Autodesk Inventor part; units mm, degrees
(part 2 of 2)
sketch "Эскиз15" plane through (8.25, 13, 36.2214) normal (0, 0, 1) x (1, 0, 0)
  line L0 (0, 4.5) -> (0, 8)
  line L1 (0, 8) -> (-1, 8)
  line L2 (0, 0) -> (0, 4.5) projected
  line L3 (0, 4.5) -> (-3, 4.5)
  line L4 (-3.75, 4.5) -> (4.75, 4.5) projected
  line L5 (-1, 8) -> (-3, 4.5)
  line L6 (-3.75, 0) -> (-12.75, 0) construction
  line L7 (-8.25, 0) -> (-8.25, 4.5) construction
  line L8 (-12.75, 4.5) -> (-3.75, 4.5) construction
  line L9 (-16.5, 4.5) -> (-16.5, 8)
  line L10 (-16.5, 8) -> (-15.5, 8)
  line L11 (-16.5, 4.5) -> (-13.5, 4.5)
  line L12 (-15.5, 8) -> (-13.5, 4.5)
  point P0 (-8.25, -13)
  dimension "d200" = 3.5
  dimension "d201" = 1
  dimension "d202" = 3
  constraints: 18 end point, 4 symmetric about line, 2 midpoint, 1 perpendicular, 1 point on line, 1 vertical
  measures "d200" distance of L0.start L0.end
  measures "d201" distance of L0.end L1.end
  measures "d202" distance of L0.start L3.end
extrude "Выдавливание14" add sketch "Эскиз15" along normal blind 25.5
sketch "Эскиз16" plane through (0, 13, 0) normal (0, 1, 0) x (1, 0, 0)
  line L0 (14.893, -63.5381) -> (15, -63.3086) projected
  arc A0 (14.893, -63.5381) -> (13, -62.9053) centre (0, -104.941) ccw projected
  line L1 (13, -62.9053) -> (13, -48.5381) projected
  line L2 (15, -48.5381) -> (13, -48.5381) projected
  line L3 (15, -48.5381) -> (15, -63.3086) projected
  arc A1 (-13, -62.9053) -> (-14.893, -63.5381) centre (0, -104.941) ccw projected
  line L4 (-15, -63.3086) -> (-14.893, -63.5381) projected
  line L5 (-15, -63.3086) -> (-15, -48.5381) projected
  line L6 (-13, -48.5381) -> (-15, -48.5381) projected
  line L7 (-13, -48.5381) -> (-13, -62.9053) projected
  line L8 (8.25, -30.9214) -> (-8.25, -30.9214) projected
  point P0 (0, 0)
extrude "Выдавливание15" add sketch "Эскиз16" along normal blind 7
sketch "Эскиз17" plane through (0, 13, 0) normal (0, 1, 0) x (1, 0, 0)
  arc A0 (13, -62.9053) -> (8.25, -61.7214) centre (0, -104.941) ccw projected
  line L0 (11.5, -48.5381) -> (11.5, -66.0381) projected
  line L1 (8.25, -36.2214) -> (8.25, -61.7214) projected
  line L2 (11.5, -48.5381) -> (13, -48.5381) projected
  line L3 (11.5, -48.5381) -> (8.25, -48.5381)
  line L4 (0, -67.941) -> (0, -60.941) construction
  line L5 (-11.5, -48.5381) -> (-8.25, -48.5381)
  arc A1 (-8.25, -61.7214) -> (-13, -62.9053) centre (0, -104.941) ccw projected
  line L6 (-8.25, -36.2214) -> (-8.25, -61.7214) projected
  line L7 (-11.5, -48.5381) -> (-11.5, -66.0381) projected
  line L8 (13, -48.5381) -> (13, -62.9053) projected
  line L9 (15, -48.5381) -> (13, -48.5381) projected
  line L10 (15, -63.3086) -> (15, -48.5381) projected
  line L11 (14.893, -63.5381) -> (15, -63.3086) projected
  arc A2 (14.893, -63.5381) -> (13, -62.9053) centre (0, -104.941) ccw projected
  line L12 (-13, -62.9053) -> (-13, -48.5381) projected
  arc A3 (-13, -62.9053) -> (-14.893, -63.5381) centre (0, -104.941) ccw projected
  line L13 (-15, -63.3086) -> (-14.893, -63.5381) projected
  line L14 (-15, -48.5381) -> (-15, -63.3086) projected
  line L15 (-13, -48.5381) -> (-15, -48.5381) projected
  line L16 (-13, -48.5381) -> (-11.5, -48.5381) projected
  line L17 (-11.5, -48.5381) -> (-13, -48.5381)
  point P0 (0, 0)
  point P1 (-13, -62.9053)
  constraints: 6 end point, 3 symmetric about line, 1 collinear, 1 perpendicular, 1 point on line
extrude "Выдавливание16" add sketch "Эскиз17" along normal blind 4.5 contours A0 L0 L2 L8 | A0 L1 L3 L0 | L5 L6 A1 L7 | L7 A1 L12 L16
extrude "Выдавливание17" add sketch "Эскиз13" along normal blind 13
chamfer "Фаска1" distance 3 angle 45 1 edges at (4.5, 13, 40)
ref_plane "РабПлоскость4" through (14.893, 35, 48.5381) normal (0, -0.0000001, -1) x (-1, 0, 0)
sketch "Эскиз18" plane through (14.893, 35, 48.5381) normal (0, -0.0000001, -1) x (-1, 0, 0)
  line L0 (29.893, 0) -> (27.893, 0) construction
  line L1 (27.893, 0) -> (27.893, -4.5) construction
  line L2 (27.893, -4.5) -> (26.393, -6) projected
  line L3 (26.393, -6) -> (26.393, -9) projected
  line L4 (26.393, -9) -> (27.893, -9) projected
  line L5 (27.893, -9) -> (27.893, -15) construction
  line L6 (27.893, -15) -> (29.893, -15) construction
  line L7 (29.893, -15) -> (29.893, 0) construction
  line L8 (1.893, -4.5) -> (1.893, 0) construction
  line L9 (1.893, 0) -> (-0.107, 0) construction
  line L10 (-0.107, 0) -> (-0.107, -15) construction
  line L11 (-0.107, -15) -> (1.893, -15) construction
  line L12 (1.893, -15) -> (1.893, -9) construction
  line L13 (1.893, -9) -> (3.393, -9) projected
  line L14 (3.393, -9) -> (3.393, -6) projected
  line L15 (3.393, -6) -> (1.893, -4.5) projected
  line L16 (27.893, -4.5) -> (27.893, -9)
  line L17 (1.893, -4.5) -> (1.893, -9) projected
  line L18 (1.893, -9) -> (1.893, -4.5)
  line L19 (3.393, -9) -> (1.893, -9) projected
  line L20 (1.893, -9) -> (3.393, -7.5)
  line L21 (3.393, -6) -> (3.393, -9) projected
  line L22 (27.893, -9) -> (26.393, -7.5)
  line L23 (26.393, -6) -> (26.393, -9) projected
  point P0 (14.893, -35)
  point P1 (26.393, -7.5)
  point P2 (3.393, -7.5)
  constraints: 8 end point, 2 midpoint, 1 collinear, 1 vertical
extrude "Выдавливание18" cut sketch "Эскиз18" against normal blind 8 contours L16 L22 L3 L2 | L17 L15 L14 L20
extrude "Выдавливание19" cut sketch "Эскиз18" against normal blind 80 contours L4 L3 L22 | L20 L14 L13
sketch "Эскиз19" plane through (0, 17.5, 0) normal (0, 1, 0) x (1, 0, 0)
  circle A0 centre (0, -40) radius 1.9 construction
  line L0 (-5.25, -61.7214) -> (-8.25, -61.7214) construction
  line L1 (-8.25, -48.5381) -> (-8.25, -61.7214) construction
  line L2 (-8.25, -48.5381) -> (-13, -48.5381) construction
  line L3 (-13, -70.3) -> (-13, -48.5381) construction
  arc A1 (-4.5, -68.2157) -> (-13, -70.3) centre (0, -104.941) ccw construction
  line L4 (-4.5, -68.2157) -> (-4.5, -54.2214) construction
  line L5 (-4.5, -54.2214) -> (4.5, -54.2214) construction
  line L6 (4.5, -54.2214) -> (4.5, -68.2157) construction
  arc A2 (13, -70.3) -> (4.5, -68.2157) centre (0, -104.941) ccw construction
  line L7 (13, -62.9053) -> (13, -70.3) construction
  line L8 (13, -48.5381) -> (13, -62.9053) construction
  line L9 (13, -48.5381) -> (8.25, -48.5381) construction
  line L10 (8.25, -61.7214) -> (8.25, -48.5381) construction
  line L11 (8.25, -61.7214) -> (5.25, -61.7214) construction
  line L12 (5.25, -61.7214) -> (5.25, -36.2214) construction
  line L13 (5.25, -36.2214) -> (8.25, -36.2214) construction
  line L14 (8.25, -36.2214) -> (8.25, -33.9214) construction
  line L15 (8.25, -33.9214) -> (-8.25, -33.9214) construction
  line L16 (-8.25, -33.9214) -> (-8.25, -36.2214) construction
  line L17 (-8.25, -36.2214) -> (-5.25, -36.2214) construction
  line L18 (-5.25, -36.2214) -> (-5.25, -61.7214) construction
  line L19 (-4.5, -61.1717) -> (-4.5, -54.2214) construction
  line L20 (-4.5, -54.2214) -> (4.5, -54.2214)
  line L21 (4.5, -33.9214) -> (-4.5, -33.9214)
  line L22 (-8.25, -33.9214) -> (8.25, -33.9214) construction
  line L23 (4.5, -54.2214) -> (4.5, -68.2157) construction
  line L24 (-4.5, -54.2214) -> (4.5, -54.2214) construction
  line L25 (2.5, -54.2214) -> (2.5, -33.9214)
  line L26 (0, -54.2214) -> (0, -33.9214) construction
  line L27 (-2.5, -54.2214) -> (-2.5, -33.9214)
  point P0 (0, 0)
  dimension "d220" = 2
  constraints: 10 end point, 2 midpoint, 2 point on line, 2 symmetric about line, 1 collinear, 1 horizontal, 1 parallel, 1 perpendicular
  measures "d220" distance between parallel lines of L6 L25
extrude "Выдавливание20" cut sketch "Эскиз19" against normal blind 3
chamfer "Фаска2" distance 2 angle 45 2 edges at (-2.5, 17.5, 44.0714) (2.5, 17.5, 44.0714)
fillet "Сопряжение1" radius 3 1 edges at (0, 13, 60.941)
